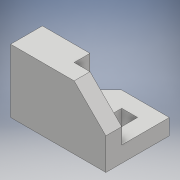
# Autodesk Inventor part: 12
Saved by Autodesk Inventor 2017 (Build 210142000, 142)
## iProperties
Part Number: 12
Material: 一般
Document SubType Name: Modeling
Designer: Brian
Density: 1 g/cm^3
Appearance: 預設
Mass: 37.5 g
Surface Area: 104.071 cm^2
Volume: 37.5 cm^3
Author: Brian
Autodesk Inventor part; units mm, degrees
ref_plane "YZ Plane" through (0, 0, 0) normal (1, 0, 0) x (0, 1, 0)
ref_plane "XZ Plane" through (0, 0, 0) normal (0, 1, 0) x (-1, 0, 0)
ref_plane "XY Plane" through (0, 0, 0) normal (0, 0, 1) x (1, 0, 0)
sketch "草圖1" plane through (0, 0, 0) normal (0, 1, 0) x (-1, 0, 0)
  line L0 (0, 0) -> (-60, 0)
  line L1 (-60, 0) -> (-60, -40)
  line L2 (-60, -40) -> (0, -40)
  line L3 (0, -40) -> (0, 0)
  dimension "d0" = 40
  dimension "d1" = 60
  constraints: 8 end point, 2 parallel, 1 horizontal, 1 perpendicular
  measures "d0" distance of L2.end L0.start
  measures "d1" distance of L1.end L2.end
extrude "擠出1" add sketch "草圖1" along normal blind 10
sketch "草圖2" plane through (0, 0, 0) normal (0, 0, 1) x (1, 0, 0)
  line L0 (0, 10) -> (60, 10) projected
  line L1 (0, 10) -> (30, 10)
  line L2 (30, 10) -> (30, 20)
  line L3 (30, 20) -> (0, 20)
  line L4 (0, 20) -> (0, 10)
  point P0 (0, 0)
  dimension "d4" = 30
  dimension "d5" = 10
  constraints: 8 end point, 2 parallel, 1 horizontal, 1 perpendicular
  measures "d4" distance of L2.end L3.end
  measures "d5" distance of L3.end L0.start
extrude "擠出2" add sketch "草圖2" against normal blind 10
sketch "草圖3" plane through (60, 0, -40) normal (0, 0, -1) x (-1, 0, 0)
  line L0 (0, 10) -> (60, 10) projected
  line L1 (0, 10) -> (30, 10)
  line L2 (30, 10) -> (30, 40)
  line L3 (30, 40) -> (0, 40)
  line L4 (0, 40) -> (0, 10)
  line L5 (60, 0) -> (60, 10) projected
  line L6 (30, 40) -> (60, 10)
  line L7 (10, 30) -> (20, 30)
  line L8 (20, 30) -> (20, 20)
  line L9 (20, 20) -> (10, 20)
  line L10 (10, 20) -> (10, 30)
  dimension "d8" = 30
  dimension "d9" = 30
  dimension "d10" = 10
  constraints: 18 end point, 4 parallel, 2 perpendicular, 1 horizontal, 3 other
  measures "d8" distance of L2.end L3.end
  measures "d9" distance of L1.end L2.end
  measures "d10" distance of L7.start L7.end
extrude "擠出3" add sketch "草圖3" against normal blind 10
chamfer "倒角1" distance 20 angle 45 1 edges at (60, 5, 0)
